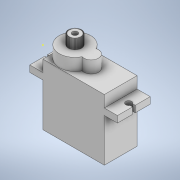
# Autodesk Inventor part: Servo Motor
Saved by Autodesk Inventor 2022 (Build 260153000, 153)
## iProperties
Created: 2023-07-22
Part Number: Servo Motor
Material: Generic
Document SubType Name: Modeling
Designer: Eric Cao
Density: 1 g/cm^3
Appearance: Default
Author: Eric Cao
Autodesk Inventor part; units mm, degrees
ref_plane "YZ Plane" through (0, 0, 0) normal (1, 0, 0) x (0, 1, 0)
ref_plane "XZ Plane" through (0, 0, 0) normal (0, 1, 0) x (-1, 0, 0)
ref_plane "XY Plane" through (0, 0, 0) normal (0, 0, 1) x (1, 0, 0)
sketch "Sketch1" plane through (0, 0, 0) normal (0, 0, 1) x (1, 0, 0)
  line L0 (0, 0) -> (22.7, 0)
  line L1 (22.7, 0) -> (22.7, 15.9)
  line L2 (22.7, 15.9) -> (27.55, 15.9)
  line L3 (27.55, 15.9) -> (27.55, 18.3)
  line L4 (27.55, 18.3) -> (22.7, 18.3)
  line L5 (22.7, 18.3) -> (22.7, 22.6)
  line L6 (22.7, 22.6) -> (0, 22.6)
  line L7 (0, 22.6) -> (0, 18.3)
  line L8 (0, 18.3) -> (-4.85, 18.3)
  line L9 (-4.85, 18.3) -> (-4.85, 15.9)
  line L10 (-4.85, 15.9) -> (0, 15.9)
  line L11 (0, 15.9) -> (0, 0)
  dimension "d0" = 22.7
  dimension "d1" = 15.9
  dimension "d2" = 4.85
  dimension "d3" = 2.4
  dimension "d4" = 4.3
  dimension "d5" = 4.85
  dimension "d6" = 15.9
  dimension "d7" = 0
  constraints: 24 end point, 9 perpendicular, 3 point on line, 1 horizontal, 1 vertical
  measures "d0" distance of L0.start L0.end
  measures "d1" distance of L0.end L1.end
  measures "d2" distance of L1.end L2.end
  measures "d3" distance of L2.end L3.end
  measures "d4" distance of L4.end L5.end
  measures "d5" distance of L7.end L8.end
  measures "d6" distance between parallel lines of L0 L10
  measures "d7" distance between parallel lines of L4 L8
extrude "Extrusion1" add sketch "Sketch1" against normal blind 12.1
sketch "Sketch2" plane through (22.7, 18.3, 0) normal (0, 1, 0) x (1, 0, 0)
  line L0 (4.85, 0) -> (4.85, 12.1) projected
  line L1 (0, 12.1) -> (4.85, 12.1) projected
  arc A0 (3.9298, 6.55) -> (3.9298, 5.55) centre (2.95, 6.05) ccw
  line L2 (3.9298, 6.55) -> (4.85, 6.55)
  line L3 (3.9298, 5.55) -> (4.85, 5.55)
  line L4 (4.85, 6.55) -> (4.85, 5.55)
  line L5 (-22.7, 0) -> (0, 0) projected
  line L6 (0, 12.1) -> (-22.7, 12.1) projected
  point P0 (-11.4934, 6.4245)
  point P1 (-12.0249, 6.05)
  dimension "d10" = 1.9
  dimension "d11" = 6.05
  dimension "d12" = 1.1
  dimension "d13" = 0.5
  dimension "d14" = 0.5
  constraints: 6 end point, 3 perpendicular, 2 point on circle, 2 point on line, 1 centre point, 1 coincident
  measures "d10" distance from line of L0 point (2.95, 6.05)
  measures "d11" distance from line of L1 point (2.95, 6.05)
  measures "d12" radius of A0
  measures "d13" distance from line of A0.centre L3
  measures "d14" distance from line of A0.centre L2
sketch "Sketch4" plane through (-4.85, 18.3, 0) normal (0, 1, 0) x (1, 0, 0)
  line L0 (0, 0) -> (0, 12.1) projected
  line L1 (0, 12.1) -> (4.85, 12.1) projected
  arc A0 (0.9202, 5.55) -> (0.9202, 6.55) centre (1.9, 6.05) ccw
  line L2 (0.9202, 6.55) -> (0, 6.55)
  line L3 (0, 0) -> (0, 12.1) projected
  line L4 (0.9202, 5.55) -> (0, 5.55)
  line L5 (0, 5.55) -> (0, 6.55)
  point P0 (4.85, 0)
  point P1 (0, 6.55)
  point P2 (0, 5.55)
  dimension "d15" = 1.9
  dimension "d16" = 6.05
  dimension "d17" = 1.1
  dimension "d18" = 0.5
  dimension "d19" = 0.5
  constraints: 6 end point, 2 point on circle, 2 point on line, 1 centre point, 1 coincident, 1 collinear, 1 horizontal, 1 parallel
  measures "d15" distance from line of L0 point (1.9, 6.05)
  measures "d16" distance from line of L1 point (1.9, 6.05)
  measures "d17" radius of A0
  measures "d18" distance from line of A0.centre L2
  measures "d19" distance from line of A0.centre L4
extrude "Extrusion2" cut sketch "Sketch2" against normal blind 12.1
extrude "Extrusion3" cut sketch "Sketch4" against normal blind 12.1
sketch "Sketch5" plane through (0, 22.6, 0) normal (0, 1, 0) x (1, 0, 0)
  line L0 (22.7, 0) -> (0, 0) projected
  arc A0 (-3.9298, 5.55) -> (-3.9298, 6.55) centre (-2.95, 6.05) ccw projected
  arc A1 (10.9958, 8.6275) -> (10.9958, 3.4725) centre (5.8, 6.05) ccw
  line L1 (0, 0) -> (0, 12.1) projected
  arc A2 (10.9958, 3.4725) -> (10.9958, 8.6275) centre (11.8, 6.05) ccw
  arc A3 (26.6298, 6.55) -> (26.6298, 5.55) centre (25.65, 6.05) ccw projected
  dimension "d24" = 6.05
  dimension "d25" = 8.75
  dimension "d26" = 6
  dimension "d27" = 5.4
  dimension "d28" = 13.85
  constraints: 4 point on circle, 2 centre point, 2 coincident, 1 tangent
  measures "d24" distance from line of L0 point (5.8, 6.05)
  measures "d25" distance of A0.centre point (5.8, 6.05)
  measures "d26" distance of point (11.8, 6.05) A1.centre
  measures "d27" diameter of A2
  measures "d28" distance of A3.centre A2.centre
extrude "Extrusion4" add sketch "Sketch5" along normal blind 4.5
sketch "Sketch6" plane through (0, 27.1, 0) normal (0, 1, 0) x (1, 0, 0)
  point P0 (0, 0)
sketch "Sketch7" plane through (0, 27.1, 0) normal (0, 1, 0) x (1, 0, 0)
  arc A0 (10.9958, 8.6275) -> (10.9958, 3.4725) centre (5.8, 6.05) ccw projected
  circle A1 centre (5.8, 6.05) radius 2.4
  point P0 (0, 0)
  point P1 (5.5563, 11.85)
  dimension "d31" = 5.8
  dimension "d32" = 4.8
  constraints: 1 centre point, 1 coincident
  measures "d31" vertical distance of A0.centre point (5.556, 11.85)
  measures "d32" diameter of A1
extrude "Extrusion5" add sketch "Sketch7" along normal blind 3.6
sketch "Sketch8" plane through (5.8, 30.7, -6.05) normal (0, 1, 0) x (1, 0, 0)
  circle A0 centre (0, 0) radius 2.4 projected
  ellipse E0 centre (0, 2.4) end of major axis (0, 2.7411) minor radius 0.1037
  ellipse E1 centre (-0.3133, 2.3795) end of major axis (-0.3578, 2.7177) minor radius 0.1037
  ellipse E2 centre (-0.6212, 2.3182) end of major axis (-0.7095, 2.6477) minor radius 0.1037
  ellipse E3 centre (-0.9184, 2.2173) end of major axis (-1.049, 2.5325) minor radius 0.1037
  ellipse E4 centre (-1.2, 2.0785) end of major axis (-1.3706, 2.3739) minor radius 0.1037
  ellipse E5 centre (-1.461, 1.904) end of major axis (-1.6687, 2.1747) minor radius 0.1037
  ellipse E6 centre (-1.6971, 1.6971) end of major axis (-1.9383, 1.9383) minor radius 0.1037
  ellipse E7 centre (-1.904, 1.461) end of major axis (-2.1747, 1.6687) minor radius 0.1037
  ellipse E8 centre (-2.0785, 1.2) end of major axis (-2.3739, 1.3706) minor radius 0.1037
  ellipse E9 centre (-2.2173, 0.9184) end of major axis (-2.5325, 1.049) minor radius 0.1037
  ellipse E10 centre (-2.3182, 0.6212) end of major axis (-2.6477, 0.7095) minor radius 0.1037
  ellipse E11 centre (-2.3795, 0.3133) end of major axis (-2.7177, 0.3578) minor radius 0.1037
  ellipse E12 centre (-2.4, 0) end of major axis (-2.7411, 0) minor radius 0.1037
  ellipse E13 centre (-2.3795, -0.3133) end of major axis (-2.7177, -0.3578) minor radius 0.1037
  ellipse E14 centre (-2.3182, -0.6212) end of major axis (-2.6477, -0.7095) minor radius 0.1037
  ellipse E15 centre (-2.2173, -0.9184) end of major axis (-2.5325, -1.049) minor radius 0.1037
  ellipse E16 centre (-2.0785, -1.2) end of major axis (-2.3739, -1.3706) minor radius 0.1037
  ellipse E17 centre (-1.904, -1.461) end of major axis (-2.1747, -1.6687) minor radius 0.1037
  ellipse E18 centre (-1.6971, -1.6971) end of major axis (-1.9383, -1.9383) minor radius 0.1037
  ellipse E19 centre (-1.461, -1.904) end of major axis (-1.6687, -2.1747) minor radius 0.1037
  ellipse E20 centre (-1.2, -2.0785) end of major axis (-1.3706, -2.3739) minor radius 0.1037
  ellipse E21 centre (-0.9184, -2.2173) end of major axis (-1.049, -2.5325) minor radius 0.1037
  ellipse E22 centre (-0.6212, -2.3182) end of major axis (-0.7095, -2.6477) minor radius 0.1037
  ellipse E23 centre (-0.3133, -2.3795) end of major axis (-0.3578, -2.7177) minor radius 0.1037
  ellipse E24 centre (0, -2.4) end of major axis (0, -2.7411) minor radius 0.1037
  ellipse E25 centre (0.3133, -2.3795) end of major axis (0.3578, -2.7177) minor radius 0.1037
  ellipse E26 centre (0.6212, -2.3182) end of major axis (0.7095, -2.6477) minor radius 0.1037
  ellipse E27 centre (0.9184, -2.2173) end of major axis (1.049, -2.5325) minor radius 0.1037
  ellipse E28 centre (1.2, -2.0785) end of major axis (1.3706, -2.3739) minor radius 0.1037
  ellipse E29 centre (1.461, -1.904) end of major axis (1.6687, -2.1747) minor radius 0.1037
  ellipse E30 centre (1.6971, -1.6971) end of major axis (1.9383, -1.9383) minor radius 0.1037
  ellipse E31 centre (1.904, -1.461) end of major axis (2.1747, -1.6687) minor radius 0.1037
  ellipse E32 centre (2.0785, -1.2) end of major axis (2.3739, -1.3706) minor radius 0.1037
  ellipse E33 centre (2.2173, -0.9184) end of major axis (2.5325, -1.049) minor radius 0.1037
  ellipse E34 centre (2.3182, -0.6212) end of major axis (2.6477, -0.7095) minor radius 0.1037
  ellipse E35 centre (2.3795, -0.3133) end of major axis (2.7177, -0.3578) minor radius 0.1037
  ellipse E36 centre (2.4, 0) end of major axis (2.7411, 0) minor radius 0.1037
  ellipse E37 centre (2.3795, 0.3133) end of major axis (2.7177, 0.3578) minor radius 0.1037
  ellipse E38 centre (2.3182, 0.6212) end of major axis (2.6477, 0.7095) minor radius 0.1037
  ellipse E39 centre (2.2173, 0.9184) end of major axis (2.5325, 1.049) minor radius 0.1037
  ellipse E40 centre (2.0785, 1.2) end of major axis (2.3739, 1.3706) minor radius 0.1037
  ellipse E41 centre (1.904, 1.461) end of major axis (2.1747, 1.6687) minor radius 0.1037
  ellipse E42 centre (1.6971, 1.6971) end of major axis (1.9383, 1.9383) minor radius 0.1037
  ellipse E43 centre (1.461, 1.904) end of major axis (1.6687, 2.1747) minor radius 0.1037
  ellipse E44 centre (1.2, 2.0785) end of major axis (1.3706, 2.3739) minor radius 0.1037
  ellipse E45 centre (0.9184, 2.2173) end of major axis (1.049, 2.5325) minor radius 0.1037
  ellipse E46 centre (0.6212, 2.3182) end of major axis (0.7095, 2.6477) minor radius 0.1037
  ellipse E47 centre (0.3133, 2.3795) end of major axis (0.3578, 2.7177) minor radius 0.1037
  point P0 (-5.8, -6.05)
  dimension "d37" = 360
  constraints: 23 centre point, 1 vertical alignment, 148 other
extrude "Extrusion6" cut sketch "Sketch8" against normal blind 3.6 contours A0 E36 | A0 E36 | E37 A0 | A0 E37 | E35 A0 | A0 E35 | E38 A0 | A0 E38 | E34 A0 | A0 E34 | E39 A0 | A0 E39 | E33 A0 | A0 E33 | E40 A0 | A0 E40 | E32 A0 | A0 E32 | E41 A0 | A0 E41 | E31 A0 | A0 E31 | E42 A0 | A0 E42 | E30 A0 | A0 E30 | E43 A0 | A0 E43 | E29 A0 | A0 E29 | E44 A0 | A0 E44 | E28 A0 | A0 E28 | E45 A0 | A0 E45 | E27 A0 | A0 E27 | E46 A0 | A0 E46 | E26 A0 | A0 E26 | E47 A0 | A0 E47 | E25 A0 | A0 E25 | E0 A0 | A0 E0 | E24 A0 | A0 E24 | E1 A0 | A0 E1 | E23 A0 | A0 E23 | E2 A0 | A0 E2 | E22 A0 | A0 E22 | E3 A0 | A0 E3 | E21 A0 | A0 E21 | E4 A0 | A0 E4 | E20 A0 | A0 E20 | E5 A0 | A0 E5 | E19 A0 | A0 E19 | E6 A0 | A0 E6 | E18 A0 | A0 E18 | E7 A0 | A0 E7 | E17 A0 | A0 E17 | E8 A0 | A0 E8 | E16 A0 | A0 E16 | E9 A0 | A0 E9 | E15 A0 | A0 E15 | E10 A0 | A0 E10 | E14 A0 | A0 E14 | E11 A0 | A0 E11 | E13 A0 | A0 E13 | E12 A0 | A0 E12
sketch "Sketch9" plane through (0, 30.7, 0) normal (0, 1, 0) x (1, 0, 0)
  arc A0 (8.1908, 5.8398) -> (8.1978, 5.9463) centre (5.8, 6.05) ccw projected
  circle A1 centre (5.8, 6.05) radius 1
  point P0 (0, 0)
  dimension "d42" = 2
  constraints: 2 coincident, 1 centre point
  measures "d42" diameter of A1
extrude "Extrusion7" cut sketch "Sketch9" against normal blind 3
body "Solid1"
